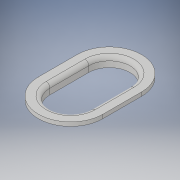
# Autodesk Inventor part: Spacer
Saved by Autodesk Inventor 2019.4 (Build 234330000, 330)
## iProperties
Created: 2020-01-27
Part Number: Spacer
Material: Generic
Document SubType Name: Modeling
Designer: Jorian Bruslind
Density: 1 g/cm^3
Appearance: Default
Author: Jorian Bruslind
Autodesk Inventor part; units mm, degrees
ref_plane "YZ Plane" through (0, 0, 0) normal (1, 0, 0) x (0, 1, 0)
ref_plane "XZ Plane" through (0, 0, 0) normal (0, 1, 0) x (-1, 0, 0)
ref_plane "XY Plane" through (0, 0, 0) normal (0, 0, 1) x (1, 0, 0)
sketch "Sketch1" plane through (0, 0, 0) normal (0, 1, 0) x (-1, 0, 0)
  line L0 (0, 0) -> (0, -15) construction
  line L1 (-9, 0) -> (-9, -15)
  line L2 (9, -15) -> (9, 0)
  arc A0 (9, 0) -> (-9, 0) centre (0, 0) ccw
  arc A1 (-9, -15) -> (9, -15) centre (0, -15) ccw
  line L3 (0, 0) -> (0, -15) construction
  line L4 (-8, 0) -> (-8, -15)
  line L5 (8, -15) -> (8, 0)
  arc A2 (8, 0) -> (-8, 0) centre (0, 0) ccw
  arc A3 (-8, -15) -> (8, -15) centre (0, -15) ccw
  point P0 (0, -7.5)
  point P1 (0, -7.5)
  dimension "d0" = 15
  dimension "d1" = 18
  dimension "d2" = 15
  dimension "d3" = 16
  constraints: 16 end point, 8 point on circle, 8 tangent, 4 centre point, 3 equal length, 2 midpoint, 1 vertical
  measures "d0" distance of L0.start L0.end
  measures "d1" diameter of A1
  measures "d2" distance of L0.start L0.end
  measures "d3" diameter of A3
extrude "Extrusion1" add sketch "Sketch1" along normal blind 3
sketch "Sketch2" plane through (0, 3, 0) normal (0, 1, 0) x (1, 0, 0)
  line L0 (0, 0) -> (0, 15) construction
  line L1 (12.5, 0) -> (12.5, 15)
  line L2 (-12.5, 15) -> (-12.5, 0)
  arc A0 (-12.5, 0) -> (12.5, 0) centre (0, 0) ccw
  arc A1 (12.5, 15) -> (-12.5, 15) centre (0, 15) ccw
  line L3 (0, 0) -> (0, 15) construction
  line L4 (8, 0) -> (8, 15)
  line L5 (-8, 15) -> (-8, 0)
  arc A2 (-8, 0) -> (8, 0) centre (0, 0) ccw
  arc A3 (8, 15) -> (-8, 15) centre (0, 15) ccw
  point P0 (0, 7.5)
  point P1 (0, 7.5)
  dimension "d6" = 15
  dimension "d7" = 25
  dimension "d8" = 15
  dimension "d9" = 16
  constraints: 16 end point, 8 point on circle, 8 tangent, 4 centre point, 3 equal length, 2 midpoint, 1 vertical
  measures "d6" distance of L0.start L0.end
  measures "d7" diameter of A1
  measures "d8" distance of L0.start L0.end
  measures "d9" diameter of A3
extrude "Extrusion2" add sketch "Sketch2" along normal mid plane 1.5
fillet "Fillet1" radius 1.5 4 edges at (0, 3.75, -23) (8, 3.75, -7.5) (0, 3.75, 8) (-8, 3.75, -7.5)
body "Solid1"
